Autodesk Fusion 360 part; units mm, degrees
note: some values were not read from the file. Set by a fixed rule: which sketch regions a step uses.
(part 7 of 59)
  spline S34 degree 5 poles (-15.0758, -14.5873) (-15.0737, -14.5855) (-15.0696, -14.582) (-15.0635, -14.5767) (-15.0553, -14.5697) (-15.045, -14.561) (-15.0349, -14.5522) (-15.0247, -14.5435) (-15.0146, -14.5347) (-15.0045, -14.526) (-14.9945, -14.5173) (-14.9845, -14.5086) (-14.9745, -14.4999) (-14.9646, -14.4912) (-14.9547, -14.4825) (-14.9448, -14.4738) (-14.935, -14.4651) (-14.9252, -14.4565) (-14.9154, -14.4478) (-14.9057, -14.4392) (-14.896, -14.4305) (-14.8863, -14.4219) (-14.8767, -14.4133) (-14.8671, -14.4047) (-14.8576, -14.3961) (-14.8481, -14.3875) (-14.8386, -14.3789) (-14.8291, -14.3703) (-14.8197, -14.3618) (-14.8104, -14.3532) (-14.801, -14.3447) (-14.7917, -14.3361) (-14.7824, -14.3276) (-14.7732, -14.3191) (-14.764, -14.3106) (-14.7549, -14.3021) (-14.7457, -14.2937) (-14.7366, -14.2852) (-14.7276, -14.2767) (-14.7186, -14.2683) (-14.7096, -14.2599) (-14.7006, -14.2515) (-14.6917, -14.2431) (-14.6829, -14.2347) (-14.674, -14.2263) (-14.6652, -14.2179) (-14.6565, -14.2096) (-14.6477, -14.2012) (-14.639, -14.1929) (-14.6304, -14.1846) (-14.6218, -14.1763) (-14.6132, -14.168) (-14.6046, -14.1597) (-14.5961, -14.1514) (-14.5877, -14.1432) (-14.5792, -14.135) (-14.5708, -14.1267) (-14.5625, -14.1185) (-14.5541, -14.1103) (-14.5459, -14.1022) (-14.5376, -14.094) (-14.5294, -14.0858) (-14.5212, -14.0777) (-14.5131, -14.0696) (-14.505, -14.0615) (-14.4969, -14.0534) (-14.4889, -14.0453) (-14.4809, -14.0373) (-14.4729, -14.0292) (-14.465, -14.0212) (-14.4571, -14.0132) (-14.4493, -14.0052) (-14.4415, -13.9972) (-14.4337, -13.9893) (-14.426, -13.9813) (-14.4183, -13.9734) (-14.4106, -13.9655) (-14.403, -13.9576) (-14.3954, -13.9497) (-14.3879, -13.9419) (-14.3804, -13.934) (-14.3729, -13.9262) (-14.3655, -13.9184) (-14.3581, -13.9106) (-14.3508, -13.9029) (-14.3435, -13.8951) (-14.3362, -13.8874) (-14.3289, -13.8797) (-14.3217, -13.872) (-14.3146, -13.8643) (-14.3075, -13.8567) (-14.3004, -13.8491) (-14.2933, -13.8414) (-14.2863, -13.8339) (-14.2794, -13.8263) (-14.2724, -13.8188) (-14.2656, -13.8112) (-14.2587, -13.8037) (-14.2519, -13.7962) (-14.2451, -13.7888) (-14.2384, -13.7813) (-14.2317, -13.7739) (-14.225, -13.7665) (-14.2184, -13.7592) (-14.2119, -13.7518) (-14.2053, -13.7445) (-14.1988, -13.7372) (-14.1924, -13.7299) (-14.1859, -13.7227) (-14.1796, -13.7154) (-14.1732, -13.7082) (-14.1669, -13.701) (-14.1607, -13.6939) (-14.1544, -13.6868) (-14.1483, -13.6796) (-14.1421, -13.6726) (-14.136, -13.6655) (-14.13, -13.6585) (-14.1239, -13.6515) (-14.118, -13.6445) (-14.112, -13.6375) (-14.1061, -13.6306) (-14.1003, -13.6237) (-14.0945, -13.6168) (-14.0887, -13.61) (-14.0829, -13.6032) (-14.0772, -13.5964) (-14.0716, -13.5896) (-14.066, -13.5829) (-14.0604, -13.5762) (-14.0549, -13.5695) (-14.0494, -13.5629) (-14.0439, -13.5563) (-14.0385, -13.5497) (-14.0332, -13.5431) (-14.0278, -13.5366) (-14.0225, -13.5301) (-14.0173, -13.5236) (-14.0121, -13.5172) (-14.0069, -13.5108) (-14.0018, -13.5044) (-13.9967, -13.4981) (-13.9917, -13.4918) (-13.9867, -13.4855) (-13.9818, -13.4793) (-13.9769, -13.4731) (-13.972, -13.4669) (-13.9672, -13.4608) (-13.9624, -13.4547) (-13.9576, -13.4486) (-13.9529, -13.4426) (-13.9483, -13.4366) (-13.9437, -13.4306) (-13.9391, -13.4247) (-13.9346, -13.4188) (-13.9301, -13.413) (-13.9257, -13.4072) (-13.9213, -13.4014) (-13.9169, -13.3957) (-13.9126, -13.39) (-13.9083, -13.3843) (-13.9041, -13.3787) (-13.8999, -13.3731) (-13.8958, -13.3676) (-13.8917, -13.3621) (-13.8876, -13.3566) (-13.8836, -13.3512) (-13.8797, -13.3458) (-13.8758, -13.3405) (-13.8719, -13.3352) (-13.8681, -13.3299) (-13.8643, -13.3247) (-13.8605, -13.3195) (-13.8568, -13.3144) (-13.8532, -13.3093) (-13.8496, -13.3043) (-13.846, -13.2993) (-13.8425, -13.2944) (-13.839, -13.2895) (-13.8356, -13.2847) (-13.8322, -13.2799) (-13.8289, -13.2751) (-13.8256, -13.2704) (-13.8224, -13.2658) (-13.8192, -13.2612) (-13.816, -13.2566) (-13.8129, -13.2521) (-13.8098, -13.2476) (-13.8068, -13.2432) (-13.8039, -13.2389) (-13.8009, -13.2346) (-13.7981, -13.2304) (-13.7952, -13.2262) (-13.7925, -13.222) (-13.7897, -13.218) (-13.787, -13.2139) (-13.7844, -13.21) (-13.7818, -13.206) (-13.7793, -13.2022) (-13.7768, -13.1984) (-13.7743, -13.1947) (-13.7719, -13.191) (-13.7696, -13.1874) (-13.7673, -13.1838) (-13.765, -13.1803) (-13.7628, -13.1769) (-13.7607, -13.1735) (-13.7586, -13.1702) (-13.7565, -13.167) (-13.7545, -13.1638) (-13.7526, -13.1607) (-13.7506, -13.1577) (-13.7488, -13.1547) (-13.747, -13.1518) (-13.7452, -13.1489) (-13.7435, -13.1462) (-13.7419, -13.1435) (-13.7403, -13.1409) (-13.7387, -13.1383) (-13.7372, -13.1358) (-13.7358, -13.1334) (-13.7344, -13.1311) (-13.733, -13.1289) (-13.7317, -13.1267) (-13.7305, -13.1246) (-13.7293, -13.1226) (-13.7282, -13.1207) (-13.7271, -13.1188) (-13.7261, -13.1171) (-13.7251, -13.1154) (-13.7242, -13.1138) (-13.7233, -13.1123) (-13.7225, -13.1109) (-13.7217, -13.1096) (-13.721, -13.1083) (-13.7204, -13.1072) (-13.7198, -13.1061) (-13.7193, -13.1052) (-13.7188, -13.1043) (-13.7184, -13.1036) (-13.718, -13.1029) (-13.7178, -13.1025) (-13.7176, -13.1022) (-13.7175, -13.102) (-13.7175, -13.1019) knots -1 -1 -1 -1 -1 -1 -0.99583333 -0.99166667 -0.9875 -0.98333333 -0.97916667 -0.975 -0.97083333 -0.96666667 -0.9625 -0.95833333 -0.95416667 -0.95 -0.94583333 -0.94166667 -0.9375 -0.93333333 -0.92916667 -0.925 -0.92083333 -0.91666667 -0.9125 -0.90833333 -0.90416667 -0.9 -0.89583333 -0.89166667 -0.8875 -0.88333333 -0.87916667 -0.875 -0.87083333 -0.86666667 -0.8625 -0.85833333 -0.85416667 -0.85 -0.84583333 -0.84166667 -0.8375 -0.83333333 -0.82916667 -0.825 -0.82083333 -0.81666667 -0.8125 -0.80833333 -0.80416667 -0.8 -0.79583333 -0.79166667 -0.7875 -0.78333333 -0.77916667 -0.775 -0.77083333 -0.76666667 -0.7625 -0.75833333 -0.75416667 -0.75 -0.74583333 -0.74166667 -0.7375 -0.73333333 -0.72916667 -0.725 -0.72083333 -0.71666667 -0.7125 -0.70833333 -0.70416667 -0.7 -0.69583333 -0.69166667 -0.6875 -0.68333333 -0.67916667 -0.675 -0.67083333 -0.66666667 -0.6625 -0.65833333 -0.65416667 -0.65 -0.64583333 -0.64166667 -0.6375 -0.63333333 -0.62916667 -0.625 -0.62083333 -0.61666667 -0.6125 -0.60833333 -0.60416667 -0.6 -0.59583333 -0.59166667 -0.5875 -0.58333333 -0.57916667 -0.575 -0.57083333 -0.56666667 -0.5625 -0.55833333 -0.55416667 -0.55 -0.54583333 -0.54166667 -0.5375 -0.53333333 -0.52916667 -0.525 -0.52083333 -0.51666667 -0.5125 -0.50833333 -0.50416667 -0.5 -0.49583333 -0.49166667 -0.4875 -0.48333333 -0.47916667 -0.475 -0.47083333 -0.46666667 -0.4625 -0.45833333 -0.45416667 -0.45 -0.44583333 -0.44166667 -0.4375 -0.43333333 -0.42916667 -0.425 -0.42083333 -0.41666667 -0.4125 -0.40833333 -0.40416667 -0.4 -0.39583333 -0.39166667 -0.3875 -0.38333333 -0.37916667 -0.375 -0.37083333 -0.36666667 -0.3625 -0.35833333 -0.35416667 -0.35 -0.34583333 -0.34166667 -0.3375 -0.33333333 -0.32916667 -0.325 -0.32083333 -0.31666667 -0.3125 -0.30833333 -0.30416667 -0.3 -0.29583333 -0.29166667 -0.2875 -0.28333333 -0.27916667 -0.275 -0.27083333 -0.26666667 -0.2625 -0.25833333 -0.25416667 -0.25 -0.24583333 -0.24166667 -0.2375 -0.23333333 -0.22916667 -0.225 -0.22083333 -0.21666667 -0.2125 -0.20833333 -0.20416667 -0.2 -0.19583333 -0.19166667 -0.1875 -0.18333333 -0.17916667 -0.175 -0.17083333 -0.16666667 -0.1625 -0.15833333 -0.15416667 -0.15 -0.14583333 -0.14166667 -0.1375 -0.13333333 -0.12916667 -0.125 -0.12083333 -0.11666667 -0.1125 -0.10833333 -0.10416667 -0.1 -0.09583333 -0.09166667 -0.0875 -0.08333333 -0.07916667 -0.075 -0.07083333 -0.06666667 -0.0625 -0.05833333 -0.05416667 -0.05 -0.04583333 -0.04166667 -0.0375 -0.03333333 -0.02916667 -0.025 -0.02083333 -0.01666667 -0.0125 -0.00833333 -0.00416667 0 0 0 0 0 0
  arc A45 (-28.4828, 8.5894) -> (-28.2972, 7.4176) centre (0, 12.5) ccw
  arc A46 (-30.8773, 9.745) -> (-30.7754, 8.7751) centre (0, 12.5) ccw
  spline S35 degree 5 poles (-30.9962, 12.0124) (-30.9936, 12.0115) (-30.9885, 12.0097) (-30.9809, 12.007) (-30.9707, 12.0034) (-30.958, 11.9989) (-30.9453, 11.9945) (-30.9327, 11.9901) (-30.9201, 11.9857) (-30.9075, 11.9813) (-30.8949, 11.977) (-30.8823, 11.9727) (-30.8698, 11.9684) (-30.8573, 11.9641) (-30.8448, 11.9599) (-30.8324, 11.9557) (-30.82, 11.9515) (-30.8076, 11.9474) (-30.7952, 11.9432) (-30.7828, 11.9391) (-30.7705, 11.9351) (-30.7582, 11.931) (-30.7459, 11.927) (-30.7337, 11.923) (-30.7215, 11.919) (-30.7093, 11.9151) (-30.6971, 11.9111) (-30.685, 11.9073) (-30.6728, 11.9034) (-30.6607, 11.8995) (-30.6487, 11.8957) (-30.6366, 11.8919) (-30.6246, 11.8882) (-30.6126, 11.8844) (-30.6007, 11.8807) (-30.5888, 11.877) (-30.5769, 11.8733) (-30.565, 11.8697) (-30.5531, 11.8661) (-30.5413, 11.8625) (-30.5295, 11.8589) (-30.5178, 11.8554) (-30.506, 11.8519) (-30.4943, 11.8484) (-30.4827, 11.8449) (-30.471, 11.8415) (-30.4594, 11.8381) (-30.4478, 11.8347) (-30.4362, 11.8313) (-30.4247, 11.828) (-30.4132, 11.8247) (-30.4017, 11.8214) (-30.3903, 11.8181) (-30.3789, 11.8149) (-30.3675, 11.8117) (-30.3562, 11.8085) (-30.3448, 11.8053) (-30.3336, 11.8022) (-30.3223, 11.7991) (-30.3111, 11.796) (-30.2999, 11.7929) (-30.2887, 11.7899) (-30.2776, 11.7869) (-30.2665, 11.7839) (-30.2554, 11.7809) (-30.2444, 11.778) (-30.2334, 11.7751) (-30.2224, 11.7722) (-30.2114, 11.7693) (-30.2005, 11.7665) (-30.1897, 11.7636) (-30.1788, 11.7609) (-30.168, 11.7581) (-30.1572, 11.7553) (-30.1465, 11.7526) (-30.1358, 11.7499) (-30.1251, 11.7472) (-30.1145, 11.7446) (-30.1038, 11.742) (-30.0933, 11.7394) (-30.0827, 11.7368) (-30.0722, 11.7342) (-30.0618, 11.7317) (-30.0513, 11.7292) (-30.0409, 11.7267) (-30.0306, 11.7242) (-30.0202, 11.7218) (-30.0099, 11.7194) (-29.9997, 11.717) (-29.9895, 11.7146) (-29.9793, 11.7123) (-29.9691, 11.71) (-29.959, 11.7077) (-29.949, 11.7054) (-29.9389, 11.7031) (-29.9289, 11.7009) (-29.919, 11.6987) (-29.909, 11.6965) (-29.8992, 11.6944) (-29.8893, 11.6922) (-29.8795, 11.6901) (-29.8697, 11.688) (-29.86, 11.686) (-29.8503, 11.6839) (-29.8407, 11.6819) (-29.8311, 11.6799) (-29.8215, 11.6779) (-29.812, 11.676) (-29.8025, 11.6741) (-29.793, 11.6721) (-29.7836, 11.6703) (-29.7742, 11.6684) (-29.7649, 11.6666) (-29.7556, 11.6647) (-29.7464, 11.6629) (-29.7372, 11.6612) (-29.728, 11.6594) (-29.7189, 11.6577) (-29.7098, 11.656) (-29.7008, 11.6543) (-29.6918, 11.6526) (-29.6828, 11.651) (-29.6739, 11.6493) (-29.6651, 11.6477) (-29.6563, 11.6462) (-29.6475, 11.6446) (-29.6388, 11.6431) (-29.6301, 11.6415) (-29.6214, 11.64) (-29.6128, 11.6386) (-29.6043, 11.6371) (-29.5958, 11.6357) (-29.5873, 11.6343) (-29.5789, 11.6329) (-29.5706, 11.6315) (-29.5623, 11.6302) (-29.554, 11.6288) (-29.5458, 11.6275) (-29.5376, 11.6262) (-29.5295, 11.625) (-29.5214, 11.6237) (-29.5134, 11.6225) (-29.5054, 11.6213) (-29.4975, 11.6201) (-29.4896, 11.6189) (-29.4818, 11.6178) (-29.474, 11.6166) (-29.4663, 11.6155) (-29.4586, 11.6144) (-29.451, 11.6134) (-29.4434, 11.6123) (-29.4359, 11.6113) (-29.4284, 11.6103) (-29.421, 11.6093) (-29.4137, 11.6083) (-29.4063, 11.6073) (-29.3991, 11.6064) (-29.3919, 11.6055) (-29.3847, 11.6046) (-29.3777, 11.6037) (-29.3706, 11.6028) (-29.3636, 11.602) (-29.3567, 11.6011) (-29.3498, 11.6003) (-29.343, 11.5995) (-29.3363, 11.5988) (-29.3296, 11.598) (-29.323, 11.5973) (-29.3164, 11.5965) (-29.3099, 11.5958) (-29.3034, 11.5951) (-29.297, 11.5945) (-29.2906, 11.5938) (-29.2844, 11.5932) (-29.2781, 11.5925) (-29.272, 11.5919) (-29.2659, 11.5913) (-29.2599, 11.5908) (-29.2539, 11.5902) (-29.248, 11.5897) (-29.2421, 11.5891) (-29.2363, 11.5886) (-29.2306, 11.5881) (-29.225, 11.5876) (-29.2194, 11.5872) (-29.2139, 11.5867) (-29.2084, 11.5863) (-29.203, 11.5859) (-29.1977, 11.5854) (-29.1925, 11.585) (-29.1873, 11.5847) (-29.1822, 11.5843) (-29.1771, 11.5839) (-29.1722, 11.5836) (-29.1673, 11.5833) (-29.1624, 11.583) (-29.1577, 11.5827) (-29.153, 11.5824) (-29.1484, 11.5821) (-29.1439, 11.5818) (-29.1394, 11.5816) (-29.135, 11.5814) (-29.1307, 11.5811) (-29.1265, 11.5809) (-29.1223, 11.5807) (-29.1183, 11.5805) (-29.1143, 11.5803) (-29.1103, 11.5802) (-29.1065, 11.58) (-29.1028, 11.5799) (-29.0991, 11.5797) (-29.0955, 11.5796) (-29.092, 11.5795) (-29.0886, 11.5794) (-29.0852, 11.5792) (-29.082, 11.5792) (-29.0788, 11.5791) (-29.0758, 11.579) (-29.0728, 11.5789) (-29.0699, 11.5789) (-29.0671, 11.5788) (-29.0644, 11.5788) (-29.0618, 11.5787) (-29.0592, 11.5787) (-29.0568, 11.5786) (-29.0545, 11.5786) (-29.0522, 11.5786) (-29.0501, 11.5786) (-29.0481, 11.5786) (-29.0461, 11.5786) (-29.0443, 11.5786) (-29.0425, 11.5786) (-29.0409, 11.5786) (-29.0394, 11.5786) (-29.038, 11.5786) (-29.0367, 11.5786) (-29.0355, 11.5786) (-29.0344, 11.5786) (-29.0334, 11.5787) (-29.0325, 11.5787) (-29.0318, 11.5787) (-29.0313, 11.5787) (-29.0309, 11.5787) (-29.0307, 11.5787) (-29.0307, 11.5787) knots -1 -1 -1 -1 -1 -1 -0.99583333 -0.99166667 -0.9875 -0.98333333 -0.97916667 -0.975 -0.97083333 -0.96666667 -0.9625 -0.95833333 -0.95416667 -0.95 -0.94583333 -0.94166667 -0.9375 -0.93333333 -0.92916667 -0.925 -0.92083333 -0.91666667 -0.9125 -0.90833333 -0.90416667 -0.9 -0.89583333 -0.89166667 -0.8875 -0.88333333 -0.87916667 -0.875 -0.87083333 -0.86666667 -0.8625 -0.85833333 -0.85416667 -0.85 -0.84583333 -0.84166667 -0.8375 -0.83333333 -0.82916667 -0.825 -0.82083333 -0.81666667 -0.8125 -0.80833333 -0.80416667 -0.8 -0.79583333 -0.79166667 -0.7875 -0.78333333 -0.77916667 -0.775 -0.77083333 -0.76666667 -0.7625 -0.75833333 -0.75416667 -0.75 -0.74583333 -0.74166667 -0.7375 -0.73333333 -0.72916667 -0.725 -0.72083333 -0.71666667 -0.7125 -0.70833333 -0.70416667 -0.7 -0.69583333 -0.69166667 -0.6875 -0.68333333 -0.67916667 -0.675 -0.67083333 -0.66666667 -0.6625 -0.65833333 -0.65416667 -0.65 -0.64583333 -0.64166667 -0.6375 -0.63333333 -0.62916667 -0.625 -0.62083333 -0.61666667 -0.6125 -0.60833333 -0.60416667 -0.6 -0.59583333 -0.59166667 -0.5875 -0.58333333 -0.57916667 -0.575 -0.57083333 -0.56666667 -0.5625 -0.55833333 -0.55416667 -0.55 -0.54583333 -0.54166667 -0.5375 -0.53333333 -0.52916667 -0.525 -0.52083333 -0.51666667 -0.5125 -0.50833333 -0.50416667 -0.5 -0.49583333 -0.49166667 -0.4875 -0.48333333 -0.47916667 -0.475 -0.47083333 -0.46666667 -0.4625 -0.45833333 -0.45416667 -0.45 -0.44583333 -0.44166667 -0.4375 -0.43333333 -0.42916667 -0.425 -0.42083333 -0.41666667 -0.4125 -0.40833333 -0.40416667 -0.4 -0.39583333 -0.39166667 -0.3875 -0.38333333 -0.37916667 -0.375 -0.37083333 -0.36666667 -0.3625 -0.35833333 -0.35416667 -0.35 -0.34583333 -0.34166667 -0.3375 -0.33333333 -0.32916667 -0.325 -0.32083333 -0.31666667 -0.3125 -0.30833333 -0.30416667 -0.3 -0.29583333 -0.29166667 -0.2875 -0.28333333 -0.27916667 -0.275 -0.27083333 -0.26666667 -0.2625 -0.25833333 -0.25416667 -0.25 -0.24583333 -0.24166667 -0.2375 -0.23333333 -0.22916667 -0.225 -0.22083333 -0.21666667 -0.2125 -0.20833333 -0.20416667 -0.2 -0.19583333 -0.19166667 -0.1875 -0.18333333 -0.17916667 -0.175 -0.17083333 -0.16666667 -0.1625 -0.15833333 -0.15416667 -0.15 -0.14583333 -0.14166667 -0.1375 -0.13333333 -0.12916667 -0.125 -0.12083333 -0.11666667 -0.1125 -0.10833333 -0.10416667 -0.1 -0.09583333 -0.09166667 -0.0875 -0.08333333 -0.07916667 -0.075 -0.07083333 -0.06666667 -0.0625 -0.05833333 -0.05416667 -0.05 -0.04583333 -0.04166667 -0.0375 -0.03333333 -0.02916667 -0.025 -0.02083333 -0.01666667 -0.0125 -0.00833333 -0.00416667 0 0 0 0 0 0
  arc A47 (-23.3609, -7.8781) -> (-22.7084, -8.6029) centre (0, 12.5) ccw
  spline S36 degree 5 poles (-26.5997, -3.4204) (-26.597, -3.4199) (-26.5917, -3.4189) (-26.5837, -3.4174) (-26.5731, -3.4154) (-26.5599, -3.413) (-26.5467, -3.4105) (-26.5335, -3.408) (-26.5204, -3.4055) (-26.5073, -3.4029) (-26.4943, -3.4004) (-26.4812, -3.3979) (-26.4682, -3.3953) (-26.4553, -3.3927) (-26.4424, -3.3902) (-26.4295, -3.3876) (-26.4166, -3.385) (-26.4038, -3.3824) (-26.391, -3.3798) (-26.3783, -3.3771) (-26.3656, -3.3745) (-26.3529, -3.3719) (-26.3403, -3.3692) (-26.3276, -3.3666) (-26.3151, -3.3639) (-26.3025, -3.3612) (-26.29, -3.3585) (-26.2776, -3.3558) (-26.2651, -3.3531) (-26.2528, -3.3504) (-26.2404, -3.3477) (-26.2281, -3.3449) (-26.2158, -3.3422) (-26.2035, -3.3394) (-26.1913, -3.3367) (-26.1792, -3.3339) (-26.167, -3.3311) (-26.1549, -3.3283) (-26.1428, -3.3255) (-26.1308, -3.3227) (-26.1188, -3.3199) (-26.1069, -3.3171) (-26.095, -3.3143) (-26.0831, -3.3115) (-26.0712, -3.3086) (-26.0594, -3.3058) (-26.0477, -3.3029) (-26.0359, -3.3001) (-26.0242, -3.2972) (-26.0126, -3.2943) (-26.001, -3.2914) (-25.9894, -3.2886) (-25.9778, -3.2857) (-25.9663, -3.2828) (-25.9549, -3.2798) (-25.9435, -3.2769) (-25.9321, -3.274) (-25.9207, -3.2711) (-25.9094, -3.2682) (-25.8982, -3.2652) (-25.8869, -3.2623) (-25.8757, -3.2593) (-25.8646, -3.2564) (-25.8535, -3.2534) (-25.8424, -3.2504) (-25.8314, -3.2475) (-25.8204, -3.2445) (-25.8094, -3.2415) (-25.7985, -3.2385) (-25.7877, -3.2355) (-25.7768, -3.2325) (-25.766, -3.2295) (-25.7553, -3.2265) (-25.7446, -3.2235) (-25.7339, -3.2205) (-25.7233, -3.2175) (-25.7127, -3.2145) (-25.7022, -3.2114) (-25.6917, -3.2084) (-25.6812, -3.2054) (-25.6708, -3.2023) (-25.6604, -3.1993) (-25.6501, -3.1963) (-25.6398, -3.1932) (-25.6296, -3.1902) (-25.6194, -3.1871) (-25.6092, -3.1841) (-25.5991, -3.181) (-25.589, -3.1779) (-25.579, -3.1749) (-25.569, -3.1718) (-25.559, -3.1688) (-25.5491, -3.1657) (-25.5393, -3.1626) (-25.5294, -3.1596) (-25.5197, -3.1565) (-25.5099, -3.1534) (-25.5003, -3.1503) (-25.4906, -3.1473) (-25.481, -3.1442) (-25.4715, -3.1411) (-25.462, -3.138) (-25.4525, -3.135) (-25.4431, -3.1319) (-25.4337, -3.1288) (-25.4244, -3.1257) (-25.4151, -3.1227) (-25.4059, -3.1196) (-25.3967, -3.1165) (-25.3876, -3.1134) (-25.3785, -3.1104) (-25.3694, -3.1073) (-25.3604, -3.1042) (-25.3515, -3.1012) (-25.3426, -3.0981) (-25.3337, -3.095) (-25.3249, -3.092) (-25.3161, -3.0889) (-25.3074, -3.0859) (-25.2988, -3.0828) (-25.2901, -3.0798) (-25.2816, -3.0767) (-25.2731, -3.0737) (-25.2646, -3.0706) (-25.2562, -3.0676) (-25.2478, -3.0645) (-25.2394, -3.0615) (-25.2312, -3.0585) (-25.2229, -3.0555) (-25.2148, -3.0524) (-25.2066, -3.0494) (-25.1986, -3.0464) (-25.1905, -3.0434) (-25.1826, -3.0404) (-25.1746, -3.0374) (-25.1668, -3.0344) (-25.1589, -3.0315) (-25.1512, -3.0285) (-25.1434, -3.0255) (-25.1358, -3.0226) (-25.1282, -3.0196) (-25.1206, -3.0166) (-25.1131, -3.0137) (-25.1056, -3.0108) (-25.0982, -3.0078) (-25.0909, -3.0049) (-25.0836, -3.002) (-25.0763, -2.9991) (-25.0691, -2.9962) (-25.062, -2.9933) (-25.0549, -2.9905) (-25.0479, -2.9876) (-25.0409, -2.9848) (-25.034, -2.9819) (-25.0271, -2.9791) (-25.0203, -2.9762) (-25.0136, -2.9734) (-25.0069, -2.9706) (-25.0002, -2.9678) (-24.9936, -2.9651) (-24.9871, -2.9623) (-24.9806, -2.9595) (-24.9742, -2.9568) (-24.9679, -2.9541) (-24.9616, -2.9514) (-24.9553, -2.9486) (-24.9492, -2.946) (-24.943, -2.9433) (-24.937, -2.9406) (-24.931, -2.938) (-24.925, -2.9353) (-24.9192, -2.9327) (-24.9133, -2.9301) (-24.9076, -2.9275) (-24.9019, -2.925) (-24.8962, -2.9224) (-24.8907, -2.9199) (-24.8852, -2.9174) (-24.8797, -2.9149) (-24.8743, -2.9124) (-24.869, -2.9099) (-24.8637, -2.9075) (-24.8585, -2.905) (-24.8534, -2.9026) (-24.8483, -2.9002) (-24.8433, -2.8979) (-24.8384, -2.8955) (-24.8335, -2.8932) (-24.8287, -2.8909) (-24.8239, -2.8886) (-24.8193, -2.8863) (-24.8147, -2.8841) (-24.8101, -2.8819) (-24.8056, -2.8797) (-24.8012, -2.8775) (-24.7969, -2.8754) (-24.7926, -2.8733) (-24.7884, -2.8712) (-24.7843, -2.8691) (-24.7802, -2.8671) (-24.7763, -2.8651) (-24.7723, -2.8631) (-24.7685, -2.8611) (-24.7647, -2.8592) (-24.761, -2.8573) (-24.7574, -2.8554) (-24.7539, -2.8536) (-24.7504, -2.8518) (-24.747, -2.85) (-24.7437, -2.8482) (-24.7404, -2.8465) (-24.7372, -2.8449) (-24.7341, -2.8432) (-24.7311, -2.8416) (-24.7282, -2.84) (-24.7253, -2.8385) (-24.7225, -2.837) (-24.7198, -2.8355) (-24.7172, -2.8341) (-24.7147, -2.8327) (-24.7122, -2.8313) (-24.7099, -2.83) (-24.7076, -2.8287) (-24.7054, -2.8275) (-24.7033, -2.8263) (-24.7012, -2.8252) (-24.6993, -2.8241) (-24.6974, -2.823) (-24.6956, -2.822) (-24.694, -2.821) (-24.6924, -2.8201) (-24.6909, -2.8193) (-24.6895, -2.8184) (-24.6881, -2.8177) (-24.6869, -2.8169) (-24.6858, -2.8163) (-24.6848, -2.8157) (-24.6838, -2.8151) (-24.683, -2.8146) (-24.6822, -2.8142) (-24.6816, -2.8138) (-24.6812, -2.8135) (-24.6809, -2.8133) (-24.6807, -2.8132) (-24.6806, -2.8132) knots -1 -1 -1 -1 -1 -1 -0.99583333 -0.99166667 -0.9875 -0.98333333 -0.97916667 -0.975 -0.97083333 -0.96666667 -0.9625 -0.95833333 -0.95416667 -0.95 -0.94583333 -0.94166667 -0.9375 -0.93333333 -0.92916667 -0.925 -0.92083333 -0.91666667 -0.9125 -0.90833333 -0.90416667 -0.9 -0.89583333 -0.89166667 -0.8875 -0.88333333 -0.87916667 -0.875 -0.87083333 -0.86666667 -0.8625 -0.85833333 -0.85416667 -0.85 -0.84583333 -0.84166667 -0.8375 -0.83333333 -0.82916667 -0.825 -0.82083333 -0.81666667 -0.8125 -0.80833333 -0.80416667 -0.8 -0.79583333 -0.79166667 -0.7875 -0.78333333 -0.77916667 -0.775 -0.77083333 -0.76666667 -0.7625 -0.75833333 -0.75416667 -0.75 -0.74583333 -0.74166667 -0.7375 -0.73333333 -0.72916667 -0.725 -0.72083333 -0.71666667 -0.7125 -0.70833333 -0.70416667 -0.7 -0.69583333 -0.69166667 -0.6875 -0.68333333 -0.67916667 -0.675 -0.67083333 -0.66666667 -0.6625 -0.65833333 -0.65416667 -0.65 -0.64583333 -0.64166667 -0.6375 -0.63333333 -0.62916667 -0.625 -0.62083333 -0.61666667 -0.6125 -0.60833333 -0.60416667 -0.6 -0.59583333 -0.59166667 -0.5875 -0.58333333 -0.57916667 -0.575 -0.57083333 -0.56666667 -0.5625 -0.55833333 -0.55416667 -0.55 -0.54583333 -0.54166667 -0.5375 -0.53333333 -0.52916667 -0.525 -0.52083333 -0.51666667 -0.5125 -0.50833333 -0.50416667 -0.5 -0.49583333 -0.49166667 -0.4875 -0.48333333 -0.47916667 -0.475 -0.47083333 -0.46666667 -0.4625 -0.45833333 -0.45416667 -0.45 -0.44583333 -0.44166667 -0.4375 -0.43333333 -0.42916667 -0.425 -0.42083333 -0.41666667 -0.4125 -0.40833333 -0.40416667 -0.4 -0.39583333 -0.39166667 -0.3875 -0.38333333 -0.37916667 -0.375 -0.37083333 -0.36666667 -0.3625 -0.35833333 -0.35416667 -0.35 -0.34583333 -0.34166667 -0.3375 -0.33333333 -0.32916667 -0.325 -0.32083333 -0.31666667 -0.3125 -0.30833333 -0.30416667 -0.3 -0.29583333 -0.29166667 -0.2875 -0.28333333 -0.27916667 -0.275 -0.27083333 -0.26666667 -0.2625 -0.25833333 -0.25416667 -0.25 -0.24583333 -0.24166667 -0.2375 -0.23333333 -0.22916667 -0.225 -0.22083333 -0.21666667 -0.2125 -0.20833333 -0.20416667 -0.2 -0.19583333 -0.19166667 -0.1875 -0.18333333 -0.17916667 -0.175 -0.17083333 -0.16666667 -0.1625 -0.15833333 -0.15416667 -0.15 -0.14583333 -0.14166667 -0.1375 -0.13333333 -0.12916667 -0.125 -0.12083333 -0.11666667 -0.1125 -0.10833333 -0.10416667 -0.1 -0.09583333 -0.09166667 -0.0875 -0.08333333 -0.07916667 -0.075 -0.07083333 -0.06666667 -0.0625 -0.05833333 -0.05416667 -0.05 -0.04583333 -0.04166667 -0.0375 -0.03333333 -0.02916667 -0.025 -0.02083333 -0.01666667 -0.0125 -0.00833333 -0.00416667 0 0 0 0 0 0
  spline S37 degree 5 poles (-30.7754, 8.7751) (-30.7728, 8.7744) (-30.7675, 8.7732) (-30.7596, 8.7713) (-30.7491, 8.7688) (-30.736, 8.7657) (-30.723, 8.7626) (-30.7099, 8.7595) (-30.6969, 8.7565) (-30.6839, 8.7534) (-30.671, 8.7504) (-30.658, 8.7475) (-30.6451, 8.7445) (-30.6323, 8.7416) (-30.6194, 8.7387) (-30.6066, 8.7358) (-30.5938, 8.733) (-30.581, 8.7301) (-30.5683, 8.7273) (-30.5556, 8.7245) (-30.5429, 8.7218) (-30.5302, 8.719) (-30.5176, 8.7163) (-30.505, 8.7136) (-30.4924, 8.7109) (-30.4799, 8.7083) (-30.4674, 8.7057) (-30.4549, 8.703) (-30.4424, 8.7005) (-30.43, 8.6979) (-30.4176, 8.6954) (-30.4053, 8.6929) (-30.3929, 8.6904) (-30.3806, 8.6879) (-30.3683, 8.6855) (-30.3561, 8.683) (-30.3439, 8.6806) (-30.3317, 8.6783) (-30.3195, 8.6759) (-30.3074, 8.6736) (-30.2953, 8.6712) (-30.2832, 8.669) (-30.2712, 8.6667) (-30.2592, 8.6644) (-30.2472, 8.6622) (-30.2353, 8.66) (-30.2233, 8.6578) (-30.2115, 8.6557) (-30.1996, 8.6536) (-30.1878, 8.6514) (-30.176, 8.6493) (-30.1643, 8.6473) (-30.1525, 8.6452) (-30.1409, 8.6432) (-30.1292, 8.6412) (-30.1176, 8.6392) (-30.106, 8.6372) (-30.0944, 8.6353) (-30.0829, 8.6334) (-30.0714, 8.6315) (-30.06, 8.6296) (-30.0486, 8.6278) (-30.0372, 8.6259) (-30.0258, 8.6241) (-30.0145, 8.6223) (-30.0032, 8.6205) (-29.992, 8.6188) (-29.9807, 8.6171) (-29.9696, 8.6154) (-29.9584, 8.6137) (-29.9473, 8.612) (-29.9362, 8.6104) (-29.9252, 8.6087) (-29.9142, 8.6071) (-29.9032, 8.6055) (-29.8923, 8.604) (-29.8814, 8.6024) (-29.8705, 8.6009) (-29.8597, 8.5994) (-29.8489, 8.5979) (-29.8382, 8.5965) (-29.8274, 8.595) (-29.8168, 8.5936) (-29.8061, 8.5922) (-29.7955, 8.5908) (-29.785, 8.5894) (-29.7744, 8.5881) (-29.764, 8.5868) (-29.7535, 8.5855) (-29.7431, 8.5842) (-29.7327, 8.5829) (-29.7224, 8.5817) (-29.7121, 8.5804) (-29.7018, 8.5792) (-29.6916, 8.578) (-29.6814, 8.5769) (-29.6713, 8.5757) (-29.6612, 8.5746) (-29.6512, 8.5735) (-29.6411, 8.5724) (-29.6312, 8.5713) (-29.6212, 8.5703) (-29.6113, 8.5692) (-29.6015, 8.5682) (-29.5917, 8.5672) (-29.5819, 8.5662) (-29.5722, 8.5652) (-29.5625, 8.5643) (-29.5529, 8.5634) (-29.5433, 8.5625) (-29.5337, 8.5616) (-29.5242, 8.5607) (-29.5147, 8.5598) (-29.5053, 8.559) (-29.4959, 8.5582) (-29.4866, 8.5574) (-29.4773, 8.5566) (-29.468, 8.5558) (-29.4588, 8.5551) (-29.4497, 8.5543) (-29.4406, 8.5536) (-29.4315, 8.5529) (-29.4225, 8.5522) (-29.4135, 8.5516) (-29.4045, 8.5509) (-29.3957, 8.5503) (-29.3868, 8.5497) (-29.378, 8.5491) (-29.3693, 8.5485) (-29.3606, 8.5479) (-29.3519, 8.5474) (-29.3433, 8.5468) (-29.3348, 8.5463) (-29.3263, 8.5458) (-29.3178, 8.5453) (-29.3094, 8.5448) (-29.301, 8.5444) (-29.2927, 8.5439) (-29.2845, 8.5435) (-29.2763, 8.5431) (-29.2681, 8.5427) (-29.26, 8.5423) (-29.2519, 8.5419) (-29.2439, 8.5416) (-29.236, 8.5412) (-29.2281, 8.5409) (-29.2202, 8.5406) (-29.2124, 8.5403) (-29.2047, 8.54) (-29.197, 8.5397) (-29.1893, 8.5395) (-29.1817, 8.5393) (-29.1742, 8.539) (-29.1667, 8.5388) (-29.1593, 8.5386) (-29.1519, 8.5384) (-29.1446, 8.5382) (-29.1374, 8.5381) (-29.1302, 8.5379) (-29.123, 8.5378) (-29.1159, 8.5377) (-29.1089, 8.5375) (-29.1019, 8.5374) (-29.095, 8.5374) (-29.0882, 8.5373) (-29.0814, 8.5372) (-29.0746, 8.5372) (-29.068, 8.5371) (-29.0613, 8.5371) (-29.0548, 8.5371) (-29.0483, 8.537) (-29.0418, 8.537) (-29.0355, 8.5371) (-29.0291, 8.5371) (-29.0229, 8.5371) (-29.0167, 8.5371) (-29.0106, 8.5372) (-29.0045, 8.5373) (-28.9985, 8.5373) (-28.9926, 8.5374) (-28.9867, 8.5375) (-28.9809, 8.5376) (-28.9752, 8.5377) (-28.9695, 8.5378) (-28.9639, 8.5379) (-28.9584, 8.538) (-28.9529, 8.5382) (-28.9475, 8.5383) (-28.9422, 8.5385) (-28.9369, 8.5386) (-28.9317, 8.5388) (-28.9266, 8.539) (-28.9215, 8.5391) (-28.9166, 8.5393) (-28.9117, 8.5395) (-28.9068, 8.5397) (-28.9021, 8.5399) (-28.8974, 8.5401) (-28.8928, 8.5403) (-28.8882, 8.5405) (-28.8838, 8.5407) (-28.8794, 8.541) (-28.8751, 8.5412) (-28.8709, 8.5414) (-28.8667, 8.5416) (-28.8626, 8.5419) (-28.8586, 8.5421) (-28.8547, 8.5423) (-28.8509, 8.5426) (-28.8472, 8.5428) (-28.8435, 8.5431) (-28.8399, 8.5433) (-28.8364, 8.5436) (-28.833, 8.5438) (-28.8297, 8.5441) (-28.8264, 8.5443) (-28.8233, 8.5445) (-28.8202, 8.5448) (-28.8172, 8.545) (-28.8144, 8.5453) (-28.8116, 8.5455) (-28.8089, 8.5457) (-28.8063, 8.546) (-28.8037, 8.5462) (-28.8013, 8.5464) (-28.799, 8.5466) (-28.7968, 8.5469) (-28.7946, 8.5471) (-28.7926, 8.5473) (-28.7907, 8.5475) (-28.7889, 8.5477) (-28.7871, 8.5478) (-28.7855, 8.548) (-28.784, 8.5482) (-28.7826, 8.5483) (-28.7813, 8.5485) (-28.7801, 8.5486) (-28.779, 8.5488) (-28.778, 8.5489) (-28.7772, 8.549) (-28.7764, 8.5491) (-28.7759, 8.5491) (-28.7756, 8.5492) (-28.7754, 8.5492) (-28.7753, 8.5492) knots -1 -1 -1 -1 -1 -1 -0.99583333 -0.99166667 -0.9875 -0.98333333 -0.97916667 -0.975 -0.97083333 -0.96666667 -0.9625 -0.95833333 -0.95416667 -0.95 -0.94583333 -0.94166667 -0.9375 -0.93333333 -0.92916667 -0.925 -0.92083333 -0.91666667 -0.9125 -0.90833333 -0.90416667 -0.9 -0.89583333 -0.89166667 -0.8875 -0.88333333 -0.87916667 -0.875 -0.87083333 -0.86666667 -0.8625 -0.85833333 -0.85416667 -0.85 -0.84583333 -0.84166667 -0.8375 -0.83333333 -0.82916667 -0.825 -0.82083333 -0.81666667 -0.8125 -0.80833333 -0.80416667 -0.8 -0.79583333 -0.79166667 -0.7875 -0.78333333 -0.77916667 -0.775 -0.77083333 -0.76666667 -0.7625 -0.75833333 -0.75416667 -0.75 -0.74583333 -0.74166667 -0.7375 -0.73333333 -0.72916667 -0.725 -0.72083333 -0.71666667 -0.7125 -0.70833333 -0.70416667 -0.7 -0.69583333 -0.69166667 -0.6875 -0.68333333 -0.67916667 -0.675 -0.67083333 -0.66666667 -0.6625 -0.65833333 -0.65416667 -0.65 -0.64583333 -0.64166667 -0.6375 -0.63333333 -0.62916667 -0.625 -0.62083333 -0.61666667 -0.6125 -0.60833333 -0.60416667 -0.6 -0.59583333 -0.59166667 -0.5875 -0.58333333 -0.57916667 -0.575 -0.57083333 -0.56666667 -0.5625 -0.55833333 -0.55416667 -0.55 -0.54583333 -0.54166667 -0.5375 -0.53333333 -0.52916667 -0.525 -0.52083333 -0.51666667 -0.5125 -0.50833333 -0.50416667 -0.5 -0.49583333 -0.49166667 -0.4875 -0.48333333 -0.47916667 -0.475 -0.47083333 -0.46666667 -0.4625 -0.45833333 -0.45416667 -0.45 -0.44583333 -0.44166667 -0.4375 -0.43333333 -0.42916667 -0.425 -0.42083333 -0.41666667 -0.4125 -0.40833333 -0.40416667 -0.4 -0.39583333 -0.39166667 -0.3875 -0.38333333 -0.37916667 -0.375 -0.37083333 -0.36666667 -0.3625 -0.35833333 -0.35416667 -0.35 -0.34583333 -0.34166667 -0.3375 -0.33333333 -0.32916667 -0.325 -0.32083333 -0.31666667 -0.3125 -0.30833333 -0.30416667 -0.3 -0.29583333 -0.29166667 -0.2875 -0.28333333 -0.27916667 -0.275 -0.27083333 -0.26666667 -0.2625 -0.25833333 -0.25416667 -0.25 -0.24583333 -0.24166667 -0.2375 -0.23333333 -0.22916667 -0.225 -0.22083333 -0.21666667 -0.2125 -0.20833333 -0.20416667 -0.2 -0.19583333 -0.19166667 -0.1875 -0.18333333 -0.17916667 -0.175 -0.17083333 -0.16666667 -0.1625 -0.15833333 -0.15416667 -0.15 -0.14583333 -0.14166667 -0.1375 -0.13333333 -0.12916667 -0.125 -0.12083333 -0.11666667 -0.1125 -0.10833333 -0.10416667 -0.1 -0.09583333 -0.09166667 -0.0875 -0.08333333 -0.07916667 -0.075 -0.07083333 -0.06666667 -0.0625 -0.05833333 -0.05416667 -0.05 -0.04583333 -0.04166667 -0.0375 -0.03333333 -0.02916667 -0.025 -0.02083333 -0.01666667 -0.0125 -0.00833333 -0.00416667 0 0 0 0 0 0
  line L99 (-26.8948, 23.4659) -> (-26.6221, 23.3547)
  arc A48 (-21.1029, -10.2084) -> (-20.3781, -10.8609) centre (0, 12.5) ccw
  spline S38 degree 5 poles (-24.0278, -3.8184) (-24.0279, -3.8185) (-24.0281, -3.8186) (-24.0283, -3.8188) (-24.0287, -3.8191) (-24.0294, -3.8195) (-24.0301, -3.82) (-24.0309, -3.8206) (-24.0317, -3.8212) (-24.0327, -3.8219) (-24.0338, -3.8227) (-24.035, -3.8235) (-24.0362, -3.8244) (-24.0375, -3.8253) (-24.0389, -3.8263) (-24.0404, -3.8274) (-24.042, -3.8286) (-24.0436, -3.8298) (-24.0453, -3.831) (-24.0471, -3.8324) (-24.049, -3.8338) (-24.051, -3.8352) (-24.053, -3.8367) (-24.0551, -3.8383) (-24.0572, -3.8399) (-24.0595, -3.8416) (-24.0618, -3.8434) (-24.0641, -3.8452) (-24.0666, -3.8471) (-24.0691, -3.849) (-24.0717, -3.851) (-24.0743, -3.853) (-24.077, -3.8551) (-24.0798, -3.8573) (-24.0826, -3.8595) (-24.0855, -3.8618) (-24.0884, -3.8641) (-24.0914, -3.8665) (-24.0945, -3.8689) (-24.0976, -3.8714) (-24.1008, -3.874) (-24.104, -3.8766) (-24.1073, -3.8792) (-24.1107, -3.8819) (-24.1141, -3.8847) (-24.1176, -3.8875) (-24.1211, -3.8904) (-24.1246, -3.8933) (-24.1283, -3.8963) (-24.1319, -3.8994) (-24.1356, -3.9024) (-24.1394, -3.9056) (-24.1432, -3.9088) (-24.1471, -3.912) (-24.151, -3.9153) (-24.155, -3.9187) (-24.159, -3.9221) (-24.1631, -3.9256) (-24.1672, -3.9291) (-24.1713, -3.9326) (-24.1755, -3.9362) (-24.1798, -3.9399) (-24.1841, -3.9436) (-24.1884, -3.9474) (-24.1928, -3.9512) (-24.1972, -3.955) (-24.2017, -3.959) (-24.2062, -3.9629) (-24.2107, -3.9669) (-24.2153, -3.971) (-24.2199, -3.9751) (-24.2246, -3.9793) (-24.2293, -3.9835) (-24.234, -3.9877) (-24.2388, -3.992) (-24.2436, -3.9964) (-24.2485, -4.0008) (-24.2534, -4.0053) (-24.2583, -4.0098) (-24.2633, -4.0143) (-24.2683, -4.0189) (-24.2733, -4.0236) (-24.2784, -4.0282) (-24.2835, -4.033) (-24.2887, -4.0378) (-24.2939, -4.0426) (-24.2991, -4.0475) (-24.3043, -4.0524) (-24.3096, -4.0574) (-24.3149, -4.0624) (-24.3203, -4.0675) (-24.3257, -4.0726) (-24.3311, -4.0778) (-24.3365, -4.083) (-24.342, -4.0882) (-24.3475, -4.0935) (-24.353, -4.0989) (-24.3586, -4.1043) (-24.3642, -4.1097) (-24.3698, -4.1152) (-24.3755, -4.1207) (-24.3812, -4.1263) (-24.3869, -4.1319) (-24.3926, -4.1376) (-24.3984, -4.1433) (-24.4042, -4.1491) (-24.41, -4.1549) (-24.4159, -4.1607) (-24.4218, -4.1666) (-24.4277, -4.1725) (-24.4336, -4.1785) (-24.4395, -4.1845) (-24.4455, -4.1906) (-24.4515, -4.1967) (-24.4576, -4.2029) (-24.4636, -4.2091) (-24.4697, -4.2153) (-24.4758, -4.2216) (-24.482, -4.2279) (-24.4881, -4.2343) (-24.4943, -4.2407) (-24.5005, -4.2472) (-24.5067, -4.2537) (-24.513, -4.2602) (-24.5192, -4.2668) (-24.5255, -4.2735) (-24.5319, -4.2801) (-24.5382, -4.2869) (-24.5446, -4.2936) (-24.5509, -4.3004) (-24.5573, -4.3073) (-24.5638, -4.3142) (-24.5702, -4.3211) (-24.5767, -4.3281) (-24.5831, -4.3351) (-24.5897, -4.3421) (-24.5962, -4.3492) (-24.6027, -4.3564) (-24.6093, -4.3636) (-24.6159, -4.3708) (-24.6225, -4.3781) (-24.6291, -4.3854) (-24.6357, -4.3927) (-24.6424, -4.4001) (-24.6491, -4.4075) (-24.6558, -4.415) (-24.6625, -4.4225) (-24.6692, -4.4301) (-24.6759, -4.4377) (-24.6827, -4.4453) (-24.6895, -4.453) (-24.6963, -4.4607) (-24.7031, -4.4685) (-24.7099, -4.4763) (-24.7168, -4.4841) (-24.7236, -4.492) (-24.7305, -4.4999) (-24.7374, -4.5079) (-24.7443, -4.5159) (-24.7512, -4.5239) (-24.7582, -4.532) (-24.7651, -4.5401) (-24.7721, -4.5483) (-24.7791, -4.5565) (-24.7861, -4.5647) (-24.7931, -4.573) (-24.8001, -4.5813) (-24.8071, -4.5897) (-24.8142, -4.5981) (-24.8212, -4.6065) (-24.8283, -4.615) (-24.8354, -4.6235) (-24.8425, -4.6321) (-24.8496, -4.6407) (-24.8568, -4.6493) (-24.8639, -4.658) (-24.8711, -4.6667) (-24.8782, -4.6754) (-24.8854, -4.6842) (-24.8926, -4.6931) (-24.8998, -4.7019) (-24.907, -4.7108) (-24.9142, -4.7198) (-24.9215, -4.7288) (-24.9287, -4.7378) (-24.936, -4.7469) (-24.9432, -4.7559) (-24.9505, -4.7651) (-24.9578, -4.7743) (-24.9651, -4.7835) (-24.9724, -4.7927) (-24.9797, -4.802) (-24.9871, -4.8113) (-24.9944, -4.8207) (-25.0017, -4.8301) (-25.0091, -4.8395) (-25.0165, -4.849) (-25.0238, -4.8585) (-25.0312, -4.8681) (-25.0386, -4.8777) (-25.046, -4.8873) (-25.0534, -4.897) (-25.0609, -4.9067) (-25.0683, -4.9164) (-25.0757, -4.9262) (-25.0832, -4.936) (-25.0906, -4.9458) (-25.0981, -4.9557) (-25.1055, -4.9657) (-25.113, -4.9756) (-25.1205, -4.9856) (-25.128, -4.9956) (-25.1355, -5.0057) (-25.143, -5.0158) (-25.1505, -5.026) (-25.158, -5.0361) (-25.1655, -5.0464) (-25.1731, -5.0566) (-25.1806, -5.0669) (-25.1881, -5.0772) (-25.1957, -5.0876) (-25.2032, -5.098) (-25.2108, -5.1084) (-25.2184, -5.1189) (-25.2259, -5.1294) (-25.2335, -5.1399) (-25.2411, -5.1505) (-25.2487, -5.1611) (-25.2563, -5.1718) (-25.2639, -5.1825) (-25.2715, -5.1932) (-25.2791, -5.2039) (-25.2867, -5.2147) (-25.2943, -5.2256) (-25.3019, -5.2364) (-25.3096, -5.2473) (-25.3172, -5.2583) (-25.3248, -5.2692) (-25.3325, -5.2802) (-25.3401, -5.2913) (-25.3477, -5.3023) (-25.3539, -5.3112) (-25.3584, -5.3179) (-25.3615, -5.3224) (-25.363, -5.3246) knots 0 0 0 0 0 0 0.00416667 0.00833333 0.0125 0.01666667 0.02083333 0.025 0.02916667 0.03333333 0.0375 0.04166667 0.04583333 0.05 0.05416667 0.05833333 0.0625 0.06666667 0.07083333 0.075 0.07916667 0.08333333 0.0875 0.09166667 0.09583333 0.1 0.10416667 0.10833333 0.1125 0.11666667 0.12083333 0.125 0.12916667 0.13333333 0.1375 0.14166667 0.14583333 0.15 0.15416667 0.15833333 0.1625 0.16666667 0.17083333 0.175 0.17916667 0.18333333 0.1875 0.19166667 0.19583333 0.2 0.20416667 0.20833333 0.2125 0.21666667 0.22083333 0.225 0.22916667 0.23333333 0.2375 0.24166667 0.24583333 0.25 0.25416667 0.25833333 0.2625 0.26666667 0.27083333 0.275 0.27916667 0.28333333 0.2875 0.29166667 0.29583333 0.3 0.30416667 0.30833333 0.3125 0.31666667 0.32083333 0.325 0.32916667 0.33333333 0.3375 0.34166667 0.34583333 0.35 0.35416667 0.35833333 0.3625 0.36666667 0.37083333 0.375 0.37916667 0.38333333 0.3875 0.39166667 0.39583333 0.4 0.40416667 0.40833333 0.4125 0.41666667 0.42083333 0.425 0.42916667 0.43333333 0.4375 0.44166667 0.44583333 0.45 0.45416667 0.45833333 0.4625 0.46666667 0.47083333 0.475 0.47916667 0.48333333 0.4875 0.49166667 0.49583333 0.5 0.50416667 0.50833333 0.5125 0.51666667 0.52083333 0.525 0.52916667 0.53333333 0.5375 0.54166667 0.54583333 0.55 0.55416667 0.55833333 0.5625 0.56666667 0.57083333 0.575 0.57916667 0.58333333 0.5875 0.59166667 0.59583333 0.6 0.60416667 0.60833333 0.6125 0.61666667 0.62083333 0.625 0.62916667 0.63333333 0.6375 0.64166667 0.64583333 0.65 0.65416667 0.65833333 0.6625 0.66666667 0.67083333 0.675 0.67916667 0.68333333 0.6875 0.69166667 0.69583333 0.7 0.70416667 0.70833333 0.7125 0.71666667 0.72083333 0.725 0.72916667 0.73333333 0.7375 0.74166667 0.74583333 0.75 0.75416667 0.75833333 0.7625 0.76666667 0.77083333 0.775 0.77916667 0.78333333 0.7875 0.79166667 0.79583333 0.8 0.80416667 0.80833333 0.8125 0.81666667 0.82083333 0.825 0.82916667 0.83333333 0.8375 0.84166667 0.84583333 0.85 0.85416667 0.85833333 0.8625 0.86666667 0.87083333 0.875 0.87916667 0.88333333 0.8875 0.89166667 0.89583333 0.9 0.90416667 0.90833333 0.9125 0.91666667 0.92083333 0.925 0.92916667 0.93333333 0.9375 0.94166667 0.94583333 0.95 0.95416667 0.95833333 0.9625 0.96666667 0.97083333 0.975 0.97916667 0.98333333 0.9875 0.99166667 0.99583333 1 1 1 1 1 1
  arc A49 (-26.6221, 23.3547) -> (-27.0473, 22.2471) centre (0, 12.5) ccw
  line L100 (-26.8955, 23.4662) -> (-26.8948, 23.4659)
  line L101 (-16.1526, 36.2836) -> (-16.318, 36.5271)
  arc A50 (-15.0758, 39.5873) -> (-15.9204, 39.0997) centre (0, 12.5) ccw
  spline S39 degree 5 poles (-13.7175, 38.1019) (-13.7175, 38.102) (-13.7176, 38.1022) (-13.7178, 38.1025) (-13.718, 38.1029) (-13.7184, 38.1036) (-13.7188, 38.1043) (-13.7193, 38.1052) (-13.7198, 38.1061) (-13.7204, 38.1072) (-13.721, 38.1083) (-13.7217, 38.1096) (-13.7225, 38.1109) (-13.7233, 38.1123) (-13.7242, 38.1138) (-13.7251, 38.1154) (-13.7261, 38.1171) (-13.7271, 38.1188) (-13.7282, 38.1207) (-13.7293, 38.1226) (-13.7305, 38.1246) (-13.7317, 38.1267) (-13.733, 38.1289) (-13.7344, 38.1311) (-13.7358, 38.1334) (-13.7372, 38.1358) (-13.7387, 38.1383) (-13.7403, 38.1409) (-13.7419, 38.1435) (-13.7435, 38.1462) (-13.7452, 38.1489) (-13.747, 38.1518) (-13.7488, 38.1547) (-13.7506, 38.1577) (-13.7526, 38.1607) (-13.7545, 38.1638) (-13.7565, 38.167) (-13.7586, 38.1702) (-13.7607, 38.1735) (-13.7628, 38.1769) (-13.765, 38.1803) (-13.7673, 38.1838) (-13.7696, 38.1874) (-13.7719, 38.191) (-13.7743, 38.1947) (-13.7768, 38.1984) (-13.7793, 38.2022) (-13.7818, 38.206) (-13.7844, 38.21) (-13.787, 38.2139) (-13.7897, 38.218) (-13.7925, 38.222) (-13.7952, 38.2262) (-13.7981, 38.2304) (-13.8009, 38.2346) (-13.8039, 38.2389) (-13.8068, 38.2432) (-13.8098, 38.2476) (-13.8129, 38.2521) (-13.816, 38.2566) (-13.8192, 38.2612) (-13.8224, 38.2658) (-13.8256, 38.2704) (-13.8289, 38.2751) (-13.8322, 38.2799) (-13.8356, 38.2847) (-13.839, 38.2895) (-13.8425, 38.2944) (-13.846, 38.2993) (-13.8496, 38.3043) (-13.8532, 38.3093) (-13.8568, 38.3144) (-13.8605, 38.3195) (-13.8643, 38.3247) (-13.8681, 38.3299) (-13.8719, 38.3352) (-13.8758, 38.3405) (-13.8797, 38.3458) (-13.8836, 38.3512) (-13.8876, 38.3566) (-13.8917, 38.3621) (-13.8958, 38.3676) (-13.8999, 38.3731) (-13.9041, 38.3787) (-13.9083, 38.3843) (-13.9126, 38.39) (-13.9169, 38.3957) (-13.9213, 38.4014) (-13.9257, 38.4072) (-13.9301, 38.413) (-13.9346, 38.4188) (-13.9391, 38.4247) (-13.9437, 38.4306) (-13.9483, 38.4366) (-13.9529, 38.4426) (-13.9576, 38.4486) (-13.9624, 38.4547) (-13.9672, 38.4608) (-13.972, 38.4669) (-13.9769, 38.4731) (-13.9818, 38.4793) (-13.9867, 38.4855) (-13.9917, 38.4918) (-13.9967, 38.4981) (-14.0018, 38.5044) (-14.0069, 38.5108) (-14.0121, 38.5172) (-14.0173, 38.5236) (-14.0225, 38.5301) (-14.0278, 38.5366) (-14.0332, 38.5431) (-14.0385, 38.5497) (-14.0439, 38.5563) (-14.0494, 38.5629) (-14.0549, 38.5695) (-14.0604, 38.5762) (-14.066, 38.5829) (-14.0716, 38.5896) (-14.0772, 38.5964) (-14.0829, 38.6032) (-14.0887, 38.61) (-14.0945, 38.6168) (-14.1003, 38.6237) (-14.1061, 38.6306) (-14.112, 38.6375) (-14.118, 38.6445) (-14.1239, 38.6515) (-14.13, 38.6585) (-14.136, 38.6655) (-14.1421, 38.6726) (-14.1483, 38.6796) (-14.1544, 38.6868) (-14.1607, 38.6939) (-14.1669, 38.701) (-14.1732, 38.7082) (-14.1796, 38.7154) (-14.1859, 38.7227) (-14.1924, 38.7299) (-14.1988, 38.7372) (-14.2053, 38.7445) (-14.2119, 38.7518) (-14.2184, 38.7592) (-14.225, 38.7665) (-14.2317, 38.7739) (-14.2384, 38.7813) (-14.2451, 38.7888) (-14.2519, 38.7962) (-14.2587, 38.8037) (-14.2656, 38.8112) (-14.2724, 38.8188) (-14.2794, 38.8263) (-14.2863, 38.8339) (-14.2933, 38.8414) (-14.3004, 38.8491) (-14.3075, 38.8567) (-14.3146, 38.8643) (-14.3217, 38.872) (-14.3289, 38.8797) (-14.3362, 38.8874) (-14.3435, 38.8951) (-14.3508, 38.9029) (-14.3581, 38.9106) (-14.3655, 38.9184) (-14.3729, 38.9262) (-14.3804, 38.934) (-14.3879, 38.9419) (-14.3954, 38.9497) (-14.403, 38.9576) (-14.4106, 38.9655) (-14.4183, 38.9734) (-14.426, 38.9813) (-14.4337, 38.9893) (-14.4415, 38.9972) (-14.4493, 39.0052) (-14.4571, 39.0132) (-14.465, 39.0212) (-14.4729, 39.0292) (-14.4809, 39.0373) (-14.4889, 39.0453) (-14.4969, 39.0534) (-14.505, 39.0615) (-14.5131, 39.0696) (-14.5212, 39.0777) (-14.5294, 39.0858) (-14.5376, 39.094) (-14.5459, 39.1022) (-14.5541, 39.1103) (-14.5625, 39.1185) (-14.5708, 39.1267) (-14.5792, 39.135) (-14.5877, 39.1432) (-14.5961, 39.1514) (-14.6046, 39.1597) (-14.6132, 39.168) (-14.6218, 39.1763) (-14.6304, 39.1846) (-14.639, 39.1929) (-14.6477, 39.2012) (-14.6565, 39.2096) (-14.6652, 39.2179) (-14.674, 39.2263) (-14.6829, 39.2347) (-14.6917, 39.2431) (-14.7006, 39.2515) (-14.7096, 39.2599) (-14.7186, 39.2683) (-14.7276, 39.2767) (-14.7366, 39.2852) (-14.7457, 39.2937) (-14.7549, 39.3021) (-14.764, 39.3106) (-14.7732, 39.3191) (-14.7824, 39.3276) (-14.7917, 39.3361) (-14.801, 39.3447) (-14.8104, 39.3532) (-14.8197, 39.3618) (-14.8291, 39.3703) (-14.8386, 39.3789) (-14.8481, 39.3875) (-14.8576, 39.3961) (-14.8671, 39.4047) (-14.8767, 39.4133) (-14.8863, 39.4219) (-14.896, 39.4305) (-14.9057, 39.4392) (-14.9154, 39.4478) (-14.9252, 39.4565) (-14.935, 39.4651) (-14.9448, 39.4738) (-14.9547, 39.4825) (-14.9646, 39.4912) (-14.9745, 39.4999) (-14.9845, 39.5086) (-14.9945, 39.5173) (-15.0045, 39.526) (-15.0146, 39.5347) (-15.0247, 39.5435) (-15.0349, 39.5522) (-15.045, 39.561) (-15.0553, 39.5697) (-15.0635, 39.5767) (-15.0696, 39.582) (-15.0737, 39.5855) (-15.0758, 39.5873) knots 0 0 0 0 0 0 0.00416667 0.00833333 0.0125 0.01666667 0.02083333 0.025 0.02916667 0.03333333 0.0375 0.04166667 0.04583333 0.05 0.05416667 0.05833333 0.0625 0.06666667 0.07083333 0.075 0.07916667 0.08333333 0.0875 0.09166667 0.09583333 0.1 0.10416667 0.10833333 0.1125 0.11666667 0.12083333 0.125 0.12916667 0.13333333 0.1375 0.14166667 0.14583333 0.15 0.15416667 0.15833333 0.1625 0.16666667 0.17083333 0.175 0.17916667 0.18333333 0.1875 0.19166667 0.19583333 0.2 0.20416667 0.20833333 0.2125 0.21666667 0.22083333 0.225 0.22916667 0.23333333 0.2375 0.24166667 0.24583333 0.25 0.25416667 0.25833333 0.2625 0.26666667 0.27083333 0.275 0.27916667 0.28333333 0.2875 0.29166667 0.29583333 0.3 0.30416667 0.30833333 0.3125 0.31666667 0.32083333 0.325 0.32916667 0.33333333 0.3375 0.34166667 0.34583333 0.35 0.35416667 0.35833333 0.3625 0.36666667 0.37083333 0.375 0.37916667 0.38333333 0.3875 0.39166667 0.39583333 0.4 0.40416667 0.40833333 0.4125 0.41666667 0.42083333 0.425 0.42916667 0.43333333 0.4375 0.44166667 0.44583333 0.45 0.45416667 0.45833333 0.4625 0.46666667 0.47083333 0.475 0.47916667 0.48333333 0.4875 0.49166667 0.49583333 0.5 0.50416667 0.50833333 0.5125 0.51666667 0.52083333 0.525 0.52916667 0.53333333 0.5375 0.54166667 0.54583333 0.55 0.55416667 0.55833333 0.5625 0.56666667 0.57083333 0.575 0.57916667 0.58333333 0.5875 0.59166667 0.59583333 0.6 0.60416667 0.60833333 0.6125 0.61666667 0.62083333 0.625 0.62916667 0.63333333 0.6375 0.64166667 0.64583333 0.65 0.65416667 0.65833333 0.6625 0.66666667 0.67083333 0.675 0.67916667 0.68333333 0.6875 0.69166667 0.69583333 0.7 0.70416667 0.70833333 0.7125 0.71666667 0.72083333 0.725 0.72916667 0.73333333 0.7375 0.74166667 0.74583333 0.75 0.75416667 0.75833333 0.7625 0.76666667 0.77083333 0.775 0.77916667 0.78333333 0.7875 0.79166667 0.79583333 0.8 0.80416667 0.80833333 0.8125 0.81666667 0.82083333 0.825 0.82916667 0.83333333 0.8375 0.84166667 0.84583333 0.85 0.85416667 0.85833333 0.8625 0.86666667 0.87083333 0.875 0.87916667 0.88333333 0.8875 0.89166667 0.89583333 0.9 0.90416667 0.90833333 0.9125 0.91666667 0.92083333 0.925 0.92916667 0.93333333 0.9375 0.94166667 0.94583333 0.95 0.95416667 0.95833333 0.9625 0.96666667 0.97083333 0.975 0.97916667 0.98333333 0.9875 0.99166667 0.99583333 1 1 1 1 1 1